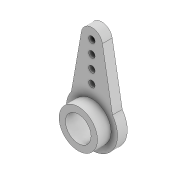
# Autodesk Inventor part: adattatore per motore
Saved by Autodesk Inventor 2022 (Build 260153000, 153)
## iProperties
Created: 2025-07-14
Part Number: adattatore per motore
Material: Generic
Document SubType Name: Modeling
Designer: 1234
Density: 1 g/cm^3
Appearance: Default
Author: 1234
Autodesk Inventor part; units mm, degrees
ref_plane "YZ Plane" through (0, 0, 0) normal (1, 0, 0) x (0, 1, 0)
ref_plane "XZ Plane" through (0, 0, 0) normal (0, 1, 0) x (-1, 0, 0)
ref_plane "XY Plane" through (0, 0, 0) normal (0, 0, 1) x (1, 0, 0)
sketch "Sketch1" plane through (0, 0, 0) normal (0, 0, 1) x (1, 0, 0)
  circle A0 centre (0, 0) radius 6
  circle A1 centre (0, 0) radius 4.5
  circle A2 centre (0, 0) radius 3
  arc A3 (2.4621, 16.9338) -> (-2.4621, 16.9338) centre (0, 16.5) ccw
  line L0 (0, 16.5) -> (0, 0) construction
  line L1 (4.8148, 3.5802) -> (2.4621, 16.9338)
  line L2 (-4.8148, 3.5802) -> (-2.4621, 16.9338)
  circle A4 centre (0, 16.5) radius 0.75
  circle A5 centre (0, 10.5) radius 0.75
  circle A6 centre (0, 7.5) radius 0.75
  circle A7 centre (0, 13.5) radius 0.75
  dimension "d0" = 12
  dimension "d1" = 9
  dimension "d2" = 6
  dimension "d3" = 5
  dimension "d4" = 16.5
  dimension "d5" = 1.5
  dimension "d6" = 1.5
  dimension "d7" = 1.5
  dimension "d8" = 1.5
  dimension "d10" = 16.5
  dimension "d11" = 13.5
  dimension "d12" = 10.5
  dimension "d13" = 7.5
  constraints: 8 centre point, 6 end point, 4 point on circle, 4 point on line, 3 coincident, 2 tangent, 1 vertical
  measures "d0" diameter of A0
  measures "d1" diameter of A1
  measures "d2" diameter of A2
  measures "d3" diameter of A3
  measures "d4" distance of point (0, 0) L0.start
  measures "d5" diameter of A4
  measures "d6" diameter of A5
  measures "d7" diameter of A6
  measures "d8" diameter of A7
  measures "d10" distance of point (0, 0) A4.centre
  measures "d11" distance of point (0, 0) A7.centre
  measures "d12" distance of point (0, 0) A5.centre
  measures "d13" distance of point (0, 0) A6.centre
extrude "Extrusion1" add sketch "Sketch1" along normal blind 2.3 contours A0 | A0 L2 A3 L1
extrude "Extrusion2" add sketch "Sketch1" along normal blind 5.5 contours A1
equation "\"d6\" = d5"
equation "\"d7\" = d5"
equation "\"d8\" = d9"
equation "\"d9\" = 1.5"
body "Solid1"
